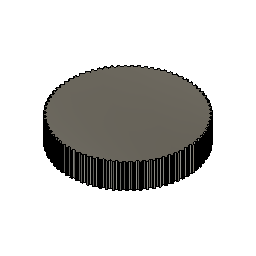
gear_77z (Autodesk Fusion 360 design; units mm, degrees)
Autodesk Fusion 360 part; units mm, degrees
sketch "Sketch1" plane through (0, 0, 0) normal (0, 0, 1) x (1, 0, 0) in component "gt2 pulley"
  circle A0 centre (0, 0) radius 24.5099 construction
  circle A1 centre (0, 0) radius 23.5059 construction
  line L0 (0, 0) -> (0, 24.5099) construction
  line L1 (0, 0) -> (0.9997, 24.4895) construction
  line L2 (0, 0) -> (1.4051, 24.4696) construction
  circle A2 centre (0, 0) radius 24.2559 construction
  arc A3 (0.3952, 24.1191) -> (0.4712, 23.8224) centre (1.3905, 24.216) ccw
  circle A4 centre (0, 0) radius 24.1059 construction
  arc A5 (0.2474, 24.2546) -> (0, 24.2559) centre (0, 0) ccw
  arc A6 (0.3952, 24.1191) -> (0.2474, 24.2546) centre (0.2459, 24.1046) ccw
  arc A7 (0.4712, 23.8224) -> (0.9588, 23.4863) centre (0.9814, 24.0408) ccw
  arc A8 (0, 24.2559) -> (-0.2474, 24.2546) centre (0, 0) ccw
  arc A9 (-0.2474, 24.2546) -> (-0.3952, 24.1191) centre (-0.2459, 24.1046) ccw
  arc A10 (-0.4712, 23.8224) -> (-0.3952, 24.1191) centre (-1.3905, 24.216) ccw
  arc A11 (-0.9589, 23.4863) -> (-0.4712, 23.8224) centre (-0.9814, 24.0408) ccw
  arc A12 (0.9588, 23.4863) -> (-0.9588, 23.4863) centre (0, 0) ccw
  point P0 (1.3905, 24.216)
  point P1 (0, 24.2559)
  dimension "d18" = 49.0197
  dimension "d19" = 2.338
  dimension "d22" = 1.004
  dimension "d24" = 0.75
  dimension "d26" = 1
  dimension "d27" = 0.15
  dimension "d28" = 0.15
  dimension "d47" = 0.555
  dimension "d52" = 3.812
  constraint coincident A0.centre A1.centre
  constraint coincident A0 L0.end
  constraint vertical L0
  constraint coincident A0 L1.end
  constraint coincident A0 L2.end
  constraint concentric A1 A2
  constraint coincident A1 A7.end
  constraint coincident L1 A7.end
  constraint coincident A2 P0
  constraint coincident L2 P0
  constraint coincident P0 A3.centre
  constraint coincident A2 P1
  constraint coincident L0 P1
  constraint concentric A2 A4
  constraint coincident P1 A5.end
  constraint coincident A4 A6.centre
  constraint coincident A3.start A6.start
  constraint tangent A3 A6
  constraint tangent A3 A7
  constraint symmetric L0 A7.end A12.end
  constraint symmetric L0 A3.start A9.end
  constraint symmetric L0 A3.end A10.start
  constraint symmetric L0 A3 A10
  constraint symmetric L0 A5.start A8.end
  constraint symmetric L0 P1 A5.end
  constraint symmetric L0 A5 A8
  constraint symmetric L0 A6 A9
  constraint symmetric L0 A7 A11
  constraint coincident A1 A11.start
  constraint tangent A1 A7
  constraint coincident L1 A7.centre
  measures "d18" diameter of A0
  measures "d19" angle of L0 L1
  measures "d22" distance of A0 A1
  measures "d24" distance of A1 A2
  measures "d26" radius of A3
  measures "d27" distance of A2 A4
  measures "d28" radius of A6
  measures "d47" radius of A7
extrude "Extrude1" add sketch "Sketch1" along normal blind 10 makes body 1
pattern_circular "C-Pattern1" count 77 over 360 about axis through (0, 0, 1.75) along (0, 0, 1) of bodies 1 makes body 2 at (-1.1717, 23.4766, 3.3333) makes body 3 at (-3.9243, 23.176, 6.6667) makes body 4 at (-5.8003, 22.779, 6.6667) makes body 5 at (-6.8266, 22.4927, 3.3333) makes body 6 at (-10.0065, 21.2696, 6.6667) makes body 7 at (-11.1481, 20.6941, 6.6667) makes body 8 at (-12.0744, 20.1676, 3.3333) makes body 9 at (-14.3623, 18.6078, 6.6667) makes body 10 at (-15.1908, 17.9378, 3.3333) makes body 11 at (-17.1948, 16.027, 6.6667) makes body 12 at (-18.8334, 14.0651, 6.6667) makes body 13 at (-19.5703, 13.0203, 6.6667) makes body 14 at (-20.8684, 10.8183, 6.6667) makes body 15 at (-21.4258, 9.6676, 6.6667) makes body 16 at (-21.8418, 8.6868, 3.3333) makes body 17 at (-22.8682, 5.438, 6.6667) makes body 18 at (-23.2353, 3.556, 6.6667) makes body 19 at (-23.3943, 2.2874, 6.6667) makes body 20 at (-23.5029, 0.3729, 6.6667) makes body 21 at (-23.4957, -0.6925, 3.3333) makes body 22 at (-23.2815, -3.2398, 6.6667) makes body 23 at (-23.0709, -4.5008, 6.6667) makes body 24 at (-22.3816, -7.1826, 6.6667) makes body 25 at (-22.0331, -8.1895, 3.3333) makes body 26 at (-20.6178, -11.2886, 6.6667) makes body 27 at (-19.629, -12.9316, 6.6667) makes body 28 at (-18.5097, -14.4885, 6.6667) makes body 29 at (-17.2672, -15.949, 6.6667) makes body 30 at (-15.9097, -17.3034, 6.6667) makes body 31 at (-14.4464, -18.5426, 6.6667) makes body 32 at (-14.1078, -18.8014, 3.3333) makes body 33 at (-12.5284, -19.8888, 3.3333) makes body 34 at (-10.1026, -21.2241, 6.6667) makes body 35 at (-8.3391, -21.9769, 6.6667) makes body 36 at (-6.52, -22.5835, 6.6667) makes body 37 at (-4.6575, -23.0398, 6.6667) makes body 38 at (-3.6087, -23.2272, 3.3333) makes body 39 at (-0.213, -23.5049, 6.6667) makes body 40 at (0.2131, -23.5049, 3.3333) makes body 41 at (2.1283, -23.4093, 3.3333) makes body 42 at (5.49, -22.8557, 6.6667) makes body 43 at (5.9035, -22.7525, 3.3333) makes body 44 at (8.5381, -21.9004, 6.6667) makes body 45 at (10.8657, -20.8438, 6.6667) makes body 46 at (11.7991, -20.33, 6.6667) makes body 47 at (14.1079, -18.8014, 6.6667) makes body 48 at (15.5935, -17.5889, 6.6667) makes body 49 at (16.9752, -16.2594, 6.6667) makes body 50 at (17.8342, -15.3123, 6.6667) makes body 51 at (19.3914, -13.2852, 6.6667) makes body 52 at (19.6291, -12.9315, 3.3333) makes body 53 at (21.0136, -10.5335, 6.6667) makes body 54 at (22.0331, -8.1894, 6.6667) makes body 55 at (22.6273, -6.3663, 6.6667) makes body 56 at (22.7921, -5.7486, 6.6667) makes body 57 at (23.361, -2.6053, 6.6667) makes body 58 at (23.4551, -1.544, 6.6667) makes body 59 at (23.4739, 1.225, 6.6667) makes body 60 at (23.3234, 2.9229, 6.6667) makes body 61 at (23.2353, 3.5561, 6.6667) makes body 62 at (22.4772, 6.8776, 6.6667) makes body 63 at (22.07, 8.0896, 6.6667) makes body 64 at (21.0611, 10.4382, 6.6667) makes body 65 at (20.8684, 10.8183, 3.3333) makes body 66 at (19.4514, 13.1973, 6.6667) makes body 67 at (17.9033, 15.2314, 6.6667) makes body 68 at (17.6242, 15.5535, 3.3333) makes body 69 at (16.2978, 16.9383, 3.3333) makes body 70 at (14.863, 18.2104, 3.3333) makes body 71 at (13.3292, 19.3612, 3.3333) makes body 72 at (10.3903, 21.0848, 6.6667) makes body 73 at (8.6371, 21.8615, 6.6667) makes body 74 at (6.8265, 22.4928, 6.6667) makes body 75 at (4.9704, 22.9743, 6.6667) makes body 76 at (3.0812, 23.303, 6.6667) makes body 77 at (1.8097, 23.4361, 6.6667)
sketch "Sketch2" plane through (0, 0, 10) normal (0, 0, 1) x (-1, 0, 0)
  arc A0 (-19.1035, -14.7291) -> (-19.1172, -14.9291) centre (-18.9991, -14.8367) ccw
  arc A1 (-19.1172, -14.9291) -> (-18.8088, -15.3159) centre (0, 0) ccw
  arc A2 (-18.8088, -15.3159) -> (-18.6107, -15.347) centre (-18.6924, -15.2212) ccw
  arc A3 (-18.3313, -15.2214) -> (-18.6107, -15.347) centre (-18.0658, -16.1855) ccw
  arc A4 (-17.7645, -15.3931) -> (-18.3313, -15.2214) centre (-18.184, -15.7565) ccw
  arc A5 (-18.9601, -13.8939) -> (-17.7645, -15.3931) centre (0, 0) ccw
  arc A6 (-18.9189, -14.4846) -> (-18.9601, -13.8939) centre (-19.4078, -14.2219) ccw
  arc A7 (-19.1035, -14.7291) -> (-18.9189, -14.4846) centre (-19.7998, -14.0113) ccw
  circle A8 centre (0, 0) radius 23.5059
  constraint concentric A1 A8
extrude "Extrude2" add sketch "Sketch2" against normal blind 10 contours A5 A8 bodies 1 2 3 4 5 6 7 8 9 10 11 12 13 14 15 16 17 18 19 20 21 22 23 24 25 26 27 28 29 30 31 32 33 34 35 36 37 38 39 40 41 42 43 44 45 46 47 48 49 50 51 52 53 54 55 56 57 58 59 60 61 62 63 64 65 66 67 68 69 70 71 72 73 74 75 76 77
extrude "Extrude4" [suppressed] in component "gt2 pulley"
pattern_circular "C-Pattern7" [suppressed] in component "gt2 pulley"
extrude "Extrude3" [suppressed] in component "gt2 pulley"
pattern_circular "C-Pattern6" [suppressed] in component "gt2 pulley"
extrude "Extrude2'" [suppressed] in component "gt2 pulley"
pattern_circular "C-Pattern5" [suppressed] in component "gt2 pulley"
extrude "Extrude1'" [suppressed] in component "gt2 pulley"
pattern_circular "C-Pattern4" [suppressed] in component "gt2 pulley"
pattern_circular "C-Pattern3" [suppressed] in component "gt2 pulley"
pattern_circular "C-Pattern2" [suppressed] in component "gt2 pulley"
pattern_circular "C-Pattern1'" [suppressed] in component "gt2 pulley"
copy_body "Body->Comp1" [suppressed] in component "Component"
copy_body "Body->Comp2" [suppressed] in component "Component'"
copy_body "Body->Comp3" [suppressed] in component "Component''"
copy_body "Body->Comp4" [suppressed] in component "Component'''"
copy_body "Body->Comp5" [suppressed] in component "Component''''"
copy_body "Body->Comp6" [suppressed] in component "Component'''''"
copy_body "Body->Comp7" [suppressed] in component "Component''''''"
copy_body "Body->Comp8" [suppressed] in component "Component'''''''"
copy_body "Body->Comp9" [suppressed] in component "Component''''''''"
copy_body "Body->Comp10" [suppressed] in component "Component'''''''''"
copy_body "Body->Comp11" [suppressed] in component "Component''''''''''"
copy_body "Body->Comp12" [suppressed] in component "Component'''''''''''"
copy_body "Body->Comp13" [suppressed] in component "Component''''''''''''"
copy_body "Body->Comp14" [suppressed] in component "Component'''''''''''''"
copy_body "Body->Comp15" [suppressed] in component "Component''''''''''''''"
copy_body "Body->Comp16" [suppressed] in component "Component'''''''''''''''"
copy_body "Body->Comp17" [suppressed] in component "Component''''''''''''''''"
copy_body "Body->Comp18" [suppressed] in component "Component'''''''''''''''''"
copy_body "Body->Comp19" [suppressed] in component "Component''''''''''''''''''"
copy_body "Body->Comp20" [suppressed] in component "Component'''''''''''''''''''"
component "gt2 pulley" placed x (1, 0, 0) y (0, 1, 0) z (0, 0, 1) at (0, 0, 0)
equation "NumTeeth = 77" comment "min 20"
equation "ToothPitch = 2 mm"
equation "PullyDia = NumTeeth * ToothPitch / PI"
equation "ToothAng = ( ( 360 / NumTeeth ) * 1 deg )"
equation "TransOffsetAngle = ToothAng * 0.2"
equation "Sholulder_Radius = 0.15 mm"
equation "Root_Radius = 0.555 mm"
equation "TransRadius = 1 mm"
equation "ToolHeight = 0.75 mm"
equation "PLD = 0.254 mm"
equation "d18 = PullyDia"
equation "d19 = ToothAng / 2"
equation "d22 = PLD + ToolHeight"
equation "d24 = ToolHeight"
equation "d26 = TransRadius"
equation "d27 = Sholulder_Radius"
equation "d31 = NumTeeth"
equation "d33 = NumTeeth"
equation "d35 = NumTeeth"
equation "d37 = NumTeeth"
equation "d41 = NumTeeth"
equation "d45 = NumTeeth"
equation "d47 = Root_Radius"
equation "d50 = NumTeeth"
